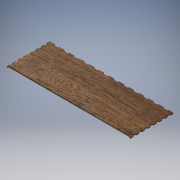
# Autodesk Inventor part: tavolaBase
Saved by Autodesk Inventor 2018.3 (Build 223284000, 284)
## iProperties
Created: 2019-03-04
Part Number: tavolaBase
Material: Generico
Document SubType Name: Modeling
Designer: AlfyPc
Density: 1 g/cm^3
Appearance: Frassino bianco - Giava
Author: AlfyPc
Autodesk Inventor part; units mm, degrees
(part 1 of 2)
ref_plane "YZ Plane" through (0, 0, 0) normal (1, 0, 0) x (0, 1, 0)
ref_plane "XZ Plane" through (0, 0, 0) normal (0, 1, 0) x (-1, 0, 0)
ref_plane "XY Plane" through (0, 0, 0) normal (0, 0, 1) x (1, 0, 0)
sketch "Schizzo1" plane through (0, 0, 0) normal (0, 0, 1) x (1, 0, 0)
  line L0 (233.5, -78.5) -> (-233.5, -78.5)
  line L1 (-233.5, -78.5) -> (-233.5, 78.5)
  line L2 (-233.5, 78.5) -> (233.5, 78.5)
  line L3 (233.5, 78.5) -> (233.5, -78.5)
  line L4 (233.5, -78.5) -> (-233.5, 78.5) construction
  line L5 (-233.5, -78.5) -> (233.5, 78.5) construction
  point P0 (0, 0)
  dimension "d0" = 467
  dimension "d1" = 157
  constraints: 12 end point, 2 midpoint, 2 parallel, 1 horizontal, 1 perpendicular
  measures "d0" distance of L0.start L0.end
  measures "d1" distance of L0.end L1.end
extrude "Estrusione1" add sketch "Schizzo1" against normal blind 4
sketch "Schizzo3" plane through (0, 0, 0) normal (0, 0, 1) x (1, 0, 0)
  line L0 (233.5, -78.5) -> (-233.5, -78.5) projected
  line L1 (233.5, 78.5) -> (233.5, -78.5) projected
  line L2 (-233.5, 78.5) -> (233.5, 78.5) projected
  line L3 (-233.5, -78.5) -> (-233.5, 78.5) projected
  line L4 (-237.5, -82.5) -> (237.5, -82.5) construction
  line L5 (237.5, -82.5) -> (237.5, 82.5) construction
  line L6 (237.5, 82.5) -> (-237.5, 82.5) construction
  line L7 (-237.5, 82.5) -> (-237.5, -82.5) construction
  line L8 (237.5, -82.5) -> (218.5, -82.5)
  line L9 (218.5, -82.5) -> (218.5, -78.5)
  line L10 (218.5, -78.5) -> (237.5, -78.5)
  line L11 (237.5, -78.5) -> (237.5, -82.5)
  line L12 (237.5, 82.5) -> (218.5, 82.5)
  line L13 (218.5, 82.5) -> (218.5, 78.5)
  line L14 (218.5, 78.5) -> (237.5, 78.5)
  line L15 (237.5, 78.5) -> (237.5, 82.5)
  line L16 (237.5, -82.5) -> (233.5, -82.5)
  line L17 (233.5, -82.5) -> (233.5, -71.5)
  line L18 (233.5, -71.5) -> (237.5, -71.5)
  line L19 (237.5, -71.5) -> (237.5, -82.5)
  line L20 (-237.5, -82.5) -> (-233.5, -82.5)
  line L21 (-233.5, -82.5) -> (-233.5, -71.5)
  line L22 (-233.5, -71.5) -> (-237.5, -71.5)
  line L23 (-237.5, -71.5) -> (-237.5, -82.5)
  line L24 (218.5, -78.5) -> (218.5, -82.5)
  line L25 (218.5, -82.5) -> (214.5, -82.5)
  line L26 (199.5, -82.5) -> (199.5, -78.5)
  line L27 (199.5, -78.5) -> (218.5, -78.5)
  line L28 (218.5, -82.5) -> (199.5, -82.5)
  line L29 (199.5, 82.5) -> (199.5, 78.5)
  line L30 (199.5, 78.5) -> (218.5, 78.5)
  line L31 (218.5, 78.5) -> (218.5, 82.5)
  line L32 (218.5, 82.5) -> (199.5, 82.5)
  line L33 (199.5, -78.5) -> (199.5, -82.5)
  line L34 (199.5, -82.5) -> (195.5, -82.5)
  line L35 (180.5, -82.5) -> (180.5, -78.5)
  line L36 (180.5, -78.5) -> (199.5, -78.5)
  line L37 (199.5, -82.5) -> (180.5, -82.5)
  line L38 (180.5, 82.5) -> (180.5, 78.5)
  line L39 (180.5, 78.5) -> (199.5, 78.5)
  line L40 (199.5, 78.5) -> (199.5, 82.5)
  line L41 (199.5, 82.5) -> (180.5, 82.5)
  line L42 (180.5, -78.5) -> (180.5, -82.5)
  line L43 (180.5, -82.5) -> (176.5, -82.5)
  line L44 (161.5, -82.5) -> (161.5, -78.5)
  line L45 (161.5, -78.5) -> (180.5, -78.5)
  line L46 (180.5, -82.5) -> (161.5, -82.5)
  line L47 (161.5, 82.5) -> (161.5, 78.5)
  line L48 (161.5, 78.5) -> (180.5, 78.5)
  line L49 (180.5, 78.5) -> (180.5, 82.5)
  line L50 (180.5, 82.5) -> (161.5, 82.5)
  line L51 (161.5, -78.5) -> (161.5, -82.5)
  line L52 (161.5, -82.5) -> (157.5, -82.5)
  line L53 (142.5, -82.5) -> (142.5, -78.5)
  line L54 (142.5, -78.5) -> (161.5, -78.5)
  line L55 (161.5, -82.5) -> (142.5, -82.5)
  line L56 (142.5, 82.5) -> (142.5, 78.5)
  line L57 (142.5, 78.5) -> (161.5, 78.5)
  line L58 (161.5, 78.5) -> (161.5, 82.5)
  line L59 (161.5, 82.5) -> (142.5, 82.5)
  line L60 (142.5, -78.5) -> (142.5, -82.5)
  line L61 (142.5, -82.5) -> (138.5, -82.5)
  line L62 (123.5, -82.5) -> (123.5, -78.5)
  line L63 (123.5, -78.5) -> (142.5, -78.5)
  line L64 (142.5, -82.5) -> (123.5, -82.5)
  line L65 (123.5, 82.5) -> (123.5, 78.5)
  line L66 (123.5, 78.5) -> (142.5, 78.5)
  line L67 (142.5, 78.5) -> (142.5, 82.5)
  line L68 (142.5, 82.5) -> (123.5, 82.5)
  line L69 (123.5, -78.5) -> (123.5, -82.5)
  line L70 (123.5, -82.5) -> (119.5, -82.5)
  line L71 (104.5, -82.5) -> (104.5, -78.5)
  line L72 (104.5, -78.5) -> (123.5, -78.5)
  line L73 (123.5, -82.5) -> (104.5, -82.5)
  line L74 (104.5, 82.5) -> (104.5, 78.5)
  line L75 (104.5, 78.5) -> (123.5, 78.5)
  line L76 (123.5, 78.5) -> (123.5, 82.5)
  line L77 (123.5, 82.5) -> (104.5, 82.5)
  line L78 (104.5, -78.5) -> (104.5, -82.5)
  line L79 (104.5, -82.5) -> (100.5, -82.5)
  line L80 (85.5, -82.5) -> (85.5, -78.5)
  line L81 (85.5, -78.5) -> (104.5, -78.5)
  line L82 (104.5, -82.5) -> (85.5, -82.5)
  line L83 (85.5, 82.5) -> (85.5, 78.5)
  line L84 (85.5, 78.5) -> (104.5, 78.5)
  line L85 (104.5, 78.5) -> (104.5, 82.5)
  line L86 (104.5, 82.5) -> (85.5, 82.5)
  line L87 (85.5, -78.5) -> (85.5, -82.5)
  line L88 (85.5, -82.5) -> (81.5, -82.5)
  line L89 (66.5, -82.5) -> (66.5, -78.5)
  line L90 (66.5, -78.5) -> (85.5, -78.5)
  line L91 (85.5, -82.5) -> (66.5, -82.5)
  line L92 (66.5, 82.5) -> (66.5, 78.5)
  line L93 (66.5, 78.5) -> (85.5, 78.5)
  line L94 (85.5, 78.5) -> (85.5, 82.5)
  line L95 (85.5, 82.5) -> (66.5, 82.5)
  line L96 (66.5, -78.5) -> (66.5, -82.5)
  line L97 (66.5, -82.5) -> (62.5, -82.5)
  line L98 (47.5, -82.5) -> (47.5, -78.5)
  line L99 (47.5, -78.5) -> (66.5, -78.5)
  line L100 (66.5, -82.5) -> (47.5, -82.5)
  line L101 (47.5, 82.5) -> (47.5, 78.5)
  line L102 (47.5, 78.5) -> (66.5, 78.5)
  line L103 (66.5, 78.5) -> (66.5, 82.5)
  line L104 (66.5, 82.5) -> (47.5, 82.5)
  line L105 (47.5, -78.5) -> (47.5, -82.5)
  line L106 (47.5, -82.5) -> (43.5, -82.5)
  line L107 (28.5, -82.5) -> (28.5, -78.5)
  line L108 (28.5, -78.5) -> (47.5, -78.5)
  line L109 (47.5, -82.5) -> (28.5, -82.5)
  line L110 (28.5, 82.5) -> (28.5, 78.5)
  line L111 (28.5, 78.5) -> (47.5, 78.5)
  line L112 (47.5, 78.5) -> (47.5, 82.5)
  line L113 (47.5, 82.5) -> (28.5, 82.5)
  line L114 (28.5, -78.5) -> (28.5, -82.5)
  line L115 (28.5, -82.5) -> (24.5, -82.5)
  line L116 (9.5, -82.5) -> (9.5, -78.5)
  line L117 (9.5, -78.5) -> (28.5, -78.5)
  line L118 (28.5, -82.5) -> (9.5, -82.5)
  line L119 (9.5, 82.5) -> (9.5, 78.5)
  line L120 (9.5, 78.5) -> (28.5, 78.5)
  line L121 (28.5, 78.5) -> (28.5, 82.5)
  line L122 (28.5, 82.5) -> (9.5, 82.5)
  line L123 (9.5, -78.5) -> (9.5, -82.5)
  line L124 (9.5, -82.5) -> (5.5, -82.5)
  line L125 (-9.5, -82.5) -> (-9.5, -78.5)
  line L126 (-9.5, -78.5) -> (9.5, -78.5)
  line L127 (9.5, -82.5) -> (-9.5, -82.5)
  line L128 (-9.5, 82.5) -> (-9.5, 78.5)
  line L129 (-9.5, 78.5) -> (9.5, 78.5)
  line L130 (9.5, 78.5) -> (9.5, 82.5)
  line L131 (9.5, 82.5) -> (-9.5, 82.5)
  line L132 (-9.5, -78.5) -> (-9.5, -82.5)
  line L133 (-9.5, -82.5) -> (-13.5, -82.5)
  line L134 (-28.5, -82.5) -> (-28.5, -78.5)
  line L135 (-28.5, -78.5) -> (-9.5, -78.5)
  line L136 (-9.5, -82.5) -> (-28.5, -82.5)
  line L137 (-28.5, 82.5) -> (-28.5, 78.5)
  line L138 (-28.5, 78.5) -> (-9.5, 78.5)
  line L139 (-9.5, 78.5) -> (-9.5, 82.5)
  line L140 (-9.5, 82.5) -> (-28.5, 82.5)
  line L141 (-28.5, -78.5) -> (-28.5, -82.5)
  line L142 (-28.5, -82.5) -> (-32.5, -82.5)
  line L143 (-47.5, -82.5) -> (-47.5, -78.5)
  line L144 (-47.5, -78.5) -> (-28.5, -78.5)
  line L145 (-28.5, -82.5) -> (-47.5, -82.5)
  line L146 (-47.5, 82.5) -> (-47.5, 78.5)
  line L147 (-47.5, 78.5) -> (-28.5, 78.5)
  line L148 (-28.5, 78.5) -> (-28.5, 82.5)
  line L149 (-28.5, 82.5) -> (-47.5, 82.5)
  line L150 (-47.5, -78.5) -> (-47.5, -82.5)
  line L151 (-47.5, -82.5) -> (-51.5, -82.5)
  line L152 (-66.5, -82.5) -> (-66.5, -78.5)
  line L153 (-66.5, -78.5) -> (-47.5, -78.5)
  line L154 (-47.5, -82.5) -> (-66.5, -82.5)
  line L155 (-66.5, 82.5) -> (-66.5, 78.5)
  line L156 (-66.5, 78.5) -> (-47.5, 78.5)
  line L157 (-47.5, 78.5) -> (-47.5, 82.5)
  line L158 (-47.5, 82.5) -> (-66.5, 82.5)
  line L159 (-66.5, -78.5) -> (-66.5, -82.5)
  line L160 (-66.5, -82.5) -> (-70.5, -82.5)
  line L161 (-85.5, -82.5) -> (-85.5, -78.5)
  line L162 (-85.5, -78.5) -> (-66.5, -78.5)
  line L163 (-66.5, -82.5) -> (-85.5, -82.5)
  line L164 (-85.5, 82.5) -> (-85.5, 78.5)
  line L165 (-85.5, 78.5) -> (-66.5, 78.5)
  line L166 (-66.5, 78.5) -> (-66.5, 82.5)
  line L167 (-66.5, 82.5) -> (-85.5, 82.5)
  line L168 (-85.5, -78.5) -> (-85.5, -82.5)
  line L169 (-85.5, -82.5) -> (-89.5, -82.5)
  line L170 (-104.5, -82.5) -> (-104.5, -78.5)
  line L171 (-104.5, -78.5) -> (-85.5, -78.5)
  line L172 (-85.5, -82.5) -> (-104.5, -82.5)
  line L173 (-104.5, 82.5) -> (-104.5, 78.5)
  line L174 (-104.5, 78.5) -> (-85.5, 78.5)
  line L175 (-85.5, 78.5) -> (-85.5, 82.5)
  line L176 (-85.5, 82.5) -> (-104.5, 82.5)
  line L177 (-104.5, -78.5) -> (-104.5, -82.5)
  line L178 (-104.5, -82.5) -> (-108.5, -82.5)
  line L179 (-123.5, -82.5) -> (-123.5, -78.5)
  line L180 (-123.5, -78.5) -> (-104.5, -78.5)
  line L181 (-104.5, -82.5) -> (-123.5, -82.5)
  line L182 (-123.5, 82.5) -> (-123.5, 78.5)
  line L183 (-123.5, 78.5) -> (-104.5, 78.5)
  line L184 (-104.5, 78.5) -> (-104.5, 82.5)
  line L185 (-104.5, 82.5) -> (-123.5, 82.5)
  line L186 (-123.5, -78.5) -> (-123.5, -82.5)
  line L187 (-123.5, -82.5) -> (-127.5, -82.5)
  line L188 (-142.5, -82.5) -> (-142.5, -78.5)
  line L189 (-142.5, -78.5) -> (-123.5, -78.5)
  line L190 (-123.5, -82.5) -> (-142.5, -82.5)
  line L191 (-142.5, 82.5) -> (-142.5, 78.5)
  line L192 (-142.5, 78.5) -> (-123.5, 78.5)
  line L193 (-123.5, 78.5) -> (-123.5, 82.5)
  line L194 (-123.5, 82.5) -> (-142.5, 82.5)
  line L195 (-142.5, -78.5) -> (-142.5, -82.5)
  line L196 (-142.5, -82.5) -> (-146.5, -82.5)
  line L197 (-161.5, -82.5) -> (-161.5, -78.5)
  line L198 (-161.5, -78.5) -> (-142.5, -78.5)
  line L199 (-142.5, -82.5) -> (-161.5, -82.5)
  line L200 (-161.5, 82.5) -> (-161.5, 78.5)
  line L201 (-161.5, 78.5) -> (-142.5, 78.5)
  line L202 (-142.5, 78.5) -> (-142.5, 82.5)
  line L203 (-142.5, 82.5) -> (-161.5, 82.5)
  line L204 (-161.5, -78.5) -> (-161.5, -82.5)
  line L205 (-161.5, -82.5) -> (-165.5, -82.5)
  line L206 (-180.5, -82.5) -> (-180.5, -78.5)
  line L207 (-180.5, -78.5) -> (-161.5, -78.5)
  line L208 (-161.5, -82.5) -> (-180.5, -82.5)
  line L209 (-180.5, 82.5) -> (-180.5, 78.5)
  line L210 (-180.5, 78.5) -> (-161.5, 78.5)
  line L211 (-161.5, 78.5) -> (-161.5, 82.5)
  line L212 (-161.5, 82.5) -> (-180.5, 82.5)
  line L213 (-180.5, -78.5) -> (-180.5, -82.5)
  line L214 (-180.5, -82.5) -> (-184.5, -82.5)
  line L215 (-199.5, -82.5) -> (-199.5, -78.5)
  line L216 (-199.5, -78.5) -> (-180.5, -78.5)
  line L217 (-180.5, -82.5) -> (-199.5, -82.5)
  line L218 (-199.5, 82.5) -> (-199.5, 78.5)
  line L219 (-199.5, 78.5) -> (-180.5, 78.5)
  line L220 (-180.5, 78.5) -> (-180.5, 82.5)
  line L221 (-180.5, 82.5) -> (-199.5, 82.5)
  line L222 (-199.5, -78.5) -> (-199.5, -82.5)
  line L223 (-199.5, -82.5) -> (-203.5, -82.5)
  line L224 (-218.5, -82.5) -> (-218.5, -78.5)
  line L225 (-218.5, -78.5) -> (-199.5, -78.5)
  line L226 (-199.5, -82.5) -> (-218.5, -82.5)
  line L227 (-218.5, 82.5) -> (-218.5, 78.5)
  line L228 (-218.5, 78.5) -> (-199.5, 78.5)
  line L229 (-199.5, 78.5) -> (-199.5, 82.5)
  line L230 (-199.5, 82.5) -> (-218.5, 82.5)
  line L231 (-218.5, -78.5) -> (-218.5, -82.5)
  line L232 (-218.5, -82.5) -> (-222.5, -82.5)
  line L233 (-237.5, -82.5) -> (-237.5, -78.5)
  line L234 (-237.5, -78.5) -> (-218.5, -78.5)
  line L235 (-218.5, -82.5) -> (-237.5, -82.5)
  line L236 (-237.5, 82.5) -> (-237.5, 78.5)
  line L237 (-237.5, 78.5) -> (-218.5, 78.5)
  line L238 (-218.5, 78.5) -> (-218.5, 82.5)
  line L239 (-218.5, 82.5) -> (-237.5, 82.5)
  line L240 (237.5, -67.5) -> (237.5, -71.5)
  line L241 (237.5, -71.5) -> (233.5, -71.5)
  line L242 (233.5, -60.5) -> (237.5, -60.5)
  line L243 (237.5, -60.5) -> (237.5, -71.5)
  line L244 (233.5, -71.5) -> (233.5, -60.5)
  line L245 (-237.5, -71.5) -> (-233.5, -71.5)
  line L246 (-233.5, -71.5) -> (-233.5, -60.5)
  line L247 (-233.5, -60.5) -> (-237.5, -60.5)
  line L248 (-237.5, -60.5) -> (-237.5, -71.5)
  line L249 (-237.5, -71.5) -> (-237.5, -67.5)
  line L250 (237.5, -56.5) -> (237.5, -60.5)
  line L251 (237.5, -60.5) -> (233.5, -60.5)
  line L252 (233.5, -49.5) -> (237.5, -49.5)
  line L253 (237.5, -49.5) -> (237.5, -60.5)
  line L254 (233.5, -60.5) -> (233.5, -49.5)
  line L255 (-237.5, -60.5) -> (-233.5, -60.5)
  line L256 (-233.5, -60.5) -> (-233.5, -49.5)
  line L257 (-233.5, -49.5) -> (-237.5, -49.5)
  line L258 (-237.5, -49.5) -> (-237.5, -60.5)
  line L259 (-237.5, -60.5) -> (-237.5, -56.5)
  line L260 (237.5, -45.5) -> (237.5, -49.5)
  line L261 (237.5, -49.5) -> (233.5, -49.5)
  line L262 (233.5, -38.5) -> (237.5, -38.5)
  line L263 (237.5, -38.5) -> (237.5, -49.5)
  line L264 (233.5, -49.5) -> (233.5, -38.5)
  line L265 (-237.5, -49.5) -> (-233.5, -49.5)
  line L266 (-233.5, -49.5) -> (-233.5, -38.5)
  line L267 (-233.5, -38.5) -> (-237.5, -38.5)
  line L268 (-237.5, -38.5) -> (-237.5, -49.5)
  line L269 (-237.5, -49.5) -> (-237.5, -45.5)
  line L270 (237.5, -34.5) -> (237.5, -38.5)
  line L271 (237.5, -38.5) -> (233.5, -38.5)
  line L272 (233.5, -27.5) -> (237.5, -27.5)
  line L273 (237.5, -27.5) -> (237.5, -38.5)
  line L274 (233.5, -38.5) -> (233.5, -27.5)
  line L275 (-237.5, -38.5) -> (-233.5, -38.5)
  line L276 (-233.5, -38.5) -> (-233.5, -27.5)
  line L277 (-233.5, -27.5) -> (-237.5, -27.5)
  line L278 (-237.5, -27.5) -> (-237.5, -38.5)
  line L279 (-237.5, -38.5) -> (-237.5, -34.5)
  line L280 (237.5, -23.5) -> (237.5, -27.5)
  line L281 (237.5, -27.5) -> (233.5, -27.5)
  line L282 (233.5, -16.5) -> (237.5, -16.5)
  line L283 (237.5, -16.5) -> (237.5, -27.5)
  line L284 (233.5, -27.5) -> (233.5, -16.5)
  line L285 (-237.5, -27.5) -> (-233.5, -27.5)
  line L286 (-233.5, -27.5) -> (-233.5, -16.5)
  line L287 (-233.5, -16.5) -> (-237.5, -16.5)
  line L288 (-237.5, -16.5) -> (-237.5, -27.5)
  line L289 (-237.5, -27.5) -> (-237.5, -23.5)
  line L290 (237.5, -12.5) -> (237.5, -16.5)
  line L291 (237.5, -16.5) -> (233.5, -16.5)
  line L292 (233.5, -5.5) -> (237.5, -5.5)
  line L293 (237.5, -5.5) -> (237.5, -16.5)
  line L294 (233.5, -16.5) -> (233.5, -5.5)
  line L295 (-237.5, -16.5) -> (-233.5, -16.5)
  line L296 (-233.5, -16.5) -> (-233.5, -5.5)
  line L297 (-233.5, -5.5) -> (-237.5, -5.5)
  line L298 (-237.5, -5.5) -> (-237.5, -16.5)
  line L299 (-237.5, -16.5) -> (-237.5, -12.5)
  line L300 (237.5, -1.5) -> (237.5, -5.5)
  line L301 (237.5, -5.5) -> (233.5, -5.5)
  line L302 (233.5, 5.5) -> (237.5, 5.5)
  line L303 (237.5, 5.5) -> (237.5, -5.5)
  line L304 (233.5, -5.5) -> (233.5, 5.5)
  line L305 (-237.5, -5.5) -> (-233.5, -5.5)
  line L306 (-233.5, -5.5) -> (-233.5, 5.5)
  line L307 (-233.5, 5.5) -> (-237.5, 5.5)
  line L308 (-237.5, 5.5) -> (-237.5, -5.5)
  line L309 (-237.5, -5.5) -> (-237.5, -1.5)
  line L310 (237.5, 9.5) -> (237.5, 5.5)
  line L311 (237.5, 5.5) -> (233.5, 5.5)
  line L312 (233.5, 16.5) -> (237.5, 16.5)
  line L313 (237.5, 16.5) -> (237.5, 5.5)
  line L314 (233.5, 5.5) -> (233.5, 16.5)
  line L315 (-237.5, 5.5) -> (-233.5, 5.5)
  line L316 (-233.5, 5.5) -> (-233.5, 16.5)
  line L317 (-233.5, 16.5) -> (-237.5, 16.5)
  line L318 (-237.5, 16.5) -> (-237.5, 5.5)
  line L319 (-237.5, 5.5) -> (-237.5, 9.5)
  line L320 (237.5, 20.5) -> (237.5, 16.5)
  line L321 (237.5, 16.5) -> (233.5, 16.5)
  line L322 (233.5, 27.5) -> (237.5, 27.5)
  line L323 (237.5, 27.5) -> (237.5, 16.5)
  line L324 (233.5, 16.5) -> (233.5, 27.5)
  line L325 (-237.5, 16.5) -> (-233.5, 16.5)
  line L326 (-233.5, 16.5) -> (-233.5, 27.5)
  line L327 (-233.5, 27.5) -> (-237.5, 27.5)
  line L328 (-237.5, 27.5) -> (-237.5, 16.5)
  line L329 (-237.5, 16.5) -> (-237.5, 20.5)
  line L330 (237.5, 31.5) -> (237.5, 27.5)
  line L331 (237.5, 27.5) -> (233.5, 27.5)
  line L332 (233.5, 38.5) -> (237.5, 38.5)
  line L333 (237.5, 38.5) -> (237.5, 27.5)
  line L334 (233.5, 27.5) -> (233.5, 38.5)
  line L335 (-237.5, 27.5) -> (-233.5, 27.5)
  line L336 (-233.5, 27.5) -> (-233.5, 38.5)
  line L337 (-233.5, 38.5) -> (-237.5, 38.5)
  line L338 (-237.5, 38.5) -> (-237.5, 27.5)
  line L339 (-237.5, 27.5) -> (-237.5, 31.5)
  line L340 (237.5, 42.5) -> (237.5, 38.5)
  line L341 (237.5, 38.5) -> (233.5, 38.5)
  line L342 (233.5, 49.5) -> (237.5, 49.5)
  line L343 (237.5, 49.5) -> (237.5, 38.5)
  line L344 (233.5, 38.5) -> (233.5, 49.5)
  line L345 (-237.5, 38.5) -> (-233.5, 38.5)
  line L346 (-233.5, 38.5) -> (-233.5, 49.5)
  line L347 (-233.5, 49.5) -> (-237.5, 49.5)
  line L348 (-237.5, 49.5) -> (-237.5, 38.5)
  line L349 (-237.5, 38.5) -> (-237.5, 42.5)
  line L350 (237.5, 53.5) -> (237.5, 49.5)
  line L351 (237.5, 49.5) -> (233.5, 49.5)
  line L352 (233.5, 60.5) -> (237.5, 60.5)
  line L353 (237.5, 60.5) -> (237.5, 49.5)
  line L354 (233.5, 49.5) -> (233.5, 60.5)
  line L355 (-237.5, 49.5) -> (-233.5, 49.5)
  line L356 (-233.5, 49.5) -> (-233.5, 60.5)
  line L357 (-233.5, 60.5) -> (-237.5, 60.5)
  line L358 (-237.5, 60.5) -> (-237.5, 49.5)
  line L359 (-237.5, 49.5) -> (-237.5, 53.5)
  line L360 (237.5, 64.5) -> (237.5, 60.5)
  line L361 (237.5, 60.5) -> (233.5, 60.5)
  line L362 (233.5, 71.5) -> (237.5, 71.5)
  line L363 (237.5, 71.5) -> (237.5, 60.5)
  line L364 (233.5, 60.5) -> (233.5, 71.5)
  line L365 (-237.5, 60.5) -> (-233.5, 60.5)
  line L366 (-233.5, 60.5) -> (-233.5, 71.5)
  line L367 (-233.5, 71.5) -> (-237.5, 71.5)
  line L368 (-237.5, 71.5) -> (-237.5, 60.5)
  line L369 (-237.5, 60.5) -> (-237.5, 64.5)
  line L370 (237.5, 75.5) -> (237.5, 71.5)
  line L371 (237.5, 71.5) -> (233.5, 71.5)
  line L372 (233.5, 82.5) -> (237.5, 82.5)
  line L373 (237.5, 82.5) -> (237.5, 71.5)
  line L374 (233.5, 71.5) -> (233.5, 82.5)
  line L375 (-237.5, 71.5) -> (-233.5, 71.5)
  line L376 (-233.5, 71.5) -> (-233.5, 82.5)
  line L377 (-233.5, 82.5) -> (-237.5, 82.5)
  line L378 (-237.5, 82.5) -> (-237.5, 71.5)
  line L379 (-237.5, 71.5) -> (-237.5, 75.5)
  point P0 (0, 0)
  point P1 (214.5, -78.5)
  point P2 (214.5, 78.5)
  point P3 (195.5, -78.5)
  point P4 (195.5, 78.5)
  point P5 (176.5, -78.5)
  point P6 (176.5, 78.5)
  point P7 (157.5, -78.5)
  point P8 (157.5, 78.5)
  point P9 (138.5, -78.5)
  point P10 (138.5, 78.5)
  point P11 (119.5, -78.5)
  point P12 (119.5, 78.5)
  point P13 (100.5, -78.5)
  point P14 (100.5, 78.5)
  point P15 (81.5, -78.5)
  point P16 (81.5, 78.5)
  point P17 (62.5, -78.5)
  point P18 (62.5, 78.5)
  point P19 (43.5, -78.5)
  point P20 (43.5, 78.5)
  point P21 (24.5, -78.5)
  point P22 (24.5, 78.5)
  point P23 (5.5, -78.5)
  point P24 (5.5, 78.5)
  point P25 (-13.5, -78.5)
  point P26 (-13.5, 78.5)
  point P27 (-32.5, -78.5)
  point P28 (-32.5, 78.5)
  point P29 (-51.5, -78.5)
  point P30 (-51.5, 78.5)
  point P31 (-70.5, -78.5)
  point P32 (-70.5, 78.5)
  point P33 (-89.5, -78.5)
  point P34 (-89.5, 78.5)
  point P35 (-108.5, -78.5)
  point P36 (-108.5, 78.5)
  point P37 (-127.5, -78.5)
  point P38 (-127.5, 78.5)
  point P39 (-146.5, -78.5)
  point P40 (-146.5, 78.5)
  point P41 (-165.5, -78.5)
  point P42 (-165.5, 78.5)
  point P43 (-184.5, -78.5)
  point P44 (-184.5, 78.5)
  point P45 (-203.5, -78.5)
  point P46 (-203.5, 78.5)
  point P47 (-222.5, -78.5)
  point P48 (-222.5, 78.5)
  point P49 (233.5, -67.5)
  point P50 (-233.5, -67.5)
  point P51 (233.5, -56.5)
  point P52 (-233.5, -56.5)
  point P53 (233.5, -45.5)
  point P54 (-233.5, -45.5)
  point P55 (233.5, -34.5)
  point P56 (-233.5, -34.5)
  point P57 (233.5, -23.5)
  point P58 (-233.5, -23.5)
  point P59 (233.5, -12.5)
  point P60 (-233.5, -12.5)
  point P61 (233.5, -1.5)
  point P62 (-233.5, -1.5)
  point P63 (233.5, 9.5)
  point P64 (-233.5, 9.5)
  point P65 (233.5, 20.5)
  point P66 (-233.5, 20.5)
  point P67 (233.5, 31.5)
  point P68 (-233.5, 31.5)
  point P69 (233.5, 42.5)
  point P70 (-233.5, 42.5)
  point P71 (233.5, 53.5)
  point P72 (-233.5, 53.5)
  point P73 (233.5, 64.5)
  point P74 (-233.5, 64.5)
  point P75 (233.5, 75.5)
  point P76 (-233.5, 75.5)
  dimension "d28" = 4
  dimension "d29" = 475
  dimension "d30" = 165
  dimension "d31" = 19
  dimension "d32" = 4
  dimension "d33" = 19
  dimension "d34" = 4
  dimension "d35" = 4
  dimension "d36" = 11
  dimension "d37" = 4
  dimension "d38" = 11
  dimension "d41" = 19
  dimension "d48" = 11
  constraints: 752 end point, 8 parallel, 5 horizontal, 4 perpendicular, 1 vertical, 805 other
  measures "d28" distance between parallel lines of L0 L4
  measures "d29" distance of L4.start L4.end
  measures "d30" distance of L4.end L5.end
  measures "d31" distance of L9.end L10.end
  measures "d32" distance of L8.end L9.end
  measures "d33" distance of L14.end L13.end
  measures "d34" distance of L13.end L12.end
  measures "d35" distance of L17.end L18.end
  measures "d36" distance of L16.end L17.end
  measures "d37" distance of L22.end L21.end
  measures "d38" distance of L21.end L20.end
  measures "d41" distance of L10.end L24.start
  measures "d48" distance of L0.start point (233.5, -67.5)
extrude "Estrusione2" add sketch "Schizzo3" against normal up to surface (4 mm away) contours L1 L18 L19 L10 | L10 L11 L8 L17 | L1 L252 L253 L250 L242 | L1 L272 L273 L270 L262 | L1 L292 L293 L290 L282 | L1 L312 L313 L310 L302 | L1 L332 L333 L330 L322 | L1 L352 L353 L350 L342 | L1 L14 L373 L370 L362 | L374 L12 L15 L14 | L2 L13 L12 L374 | L2 L38 L41 L29 | L2 L56 L59 L47 | L2 L74 L77 L65 | L2 L92 L95 L83 | L234 L23 L22 L3 | L21 L20 L23 L234 | L2 L110 L113 L101 | L247 L258 L257 L3 | L2 L128 L131 L119 | L267 L278 L277 L3 | L2 L146 L149 L137 | L287 L298 L297 L3 | L2 L164 L167 L155 | L307 L318 L317 L3 | L2 L182 L185 L173 | L327 L338 L337 L3 | L2 L200 L203 L191 | L347 L358 L357 L3 | L2 L218 L221 L209 | L367 L378 L237 L3 | L2 L376 L239 L227 | L237 L236 L239 L376
sketch "Schizzo4" plane through (0, 0, 0) normal (0, 0, 1) x (1, 0, 0)
  circle A0 centre (29.075, -39.395) radius 1.5
  circle A1 centre (29.075, 41.885) radius 1.5
  circle A2 centre (-135.39, -38.76) radius 1.5
  circle A3 centre (-173.97, 42.5) radius 1.375
  circle A4 centre (-222.97, 42.5) radius 1.375
  circle A5 centre (-173.97, -15.5) radius 1.375
  circle A6 centre (-222.97, -15.5) radius 1.375
  point P0 (0, 0)
extrude "Estrusione3" cut sketch "Schizzo4" against normal blind 10
sketch "Schizzo5" plane through (0, 0, 0) normal (0, 0, 1) x (1, 0, 0)
  line L0 (-55.35, 78.5) -> (-58.65, 78.5) projected
  line L1 (-233.5, -64.35) -> (-233.5, -67.65) projected
  line L2 (-233.5, -71.5) -> (-233.5, -60.5) construction
  line L3 (-233.5, -66) -> (-220.5, -66) construction
  circle A0 centre (-220.5, -66) radius 1.65
  line L4 (-66.5, 78.5) -> (-47.5, 78.5) construction
  line L5 (-57, 78.5) -> (-57, 65.5) construction
  circle A1 centre (-57, 65.5) radius 1.65
  line L6 (233.5, -67.65) -> (233.5, -64.35) projected
  line L7 (233.5, -60.5) -> (233.5, -71.5) projected
  line L8 (233.5, -66) -> (220.5, -66) construction
  circle A2 centre (220.5, -66) radius 1.65
  dimension "d75" = 13
  dimension "d76" = 3.3
  dimension "d77" = 13
  dimension "d78" = 3.3
  dimension "d79" = 13
  dimension "d80" = 3.3
  constraints: 6 end point, 3 centre point, 3 coincident, 3 midpoint, 1 horizontal, 1 perpendicular, 1 vertical
  measures "d75" distance of L3.start L3.end
  measures "d76" diameter of A0
  measures "d77" distance of L5.start L5.end
  measures "d78" diameter of A1
  measures "d79" distance of L8.start L8.end
  measures "d80" diameter of A2
extrude "Estrusione4" cut sketch "Schizzo5" against normal blind 10
sketch "Schizzo6" plane through (0, 0, 0) normal (0, 0, 1) x (1, 0, 0)
  line L0 (-139.4893, -62.5844) -> (-76.5866, -62.5844) construction
  line L1 (-76.5866, -62.5844) -> (-76.5866, -76.1722) construction
  line L2 (-76.5866, -76.1722) -> (-139.4893, -76.1722) construction
  line L3 (-139.4893, -76.1722) -> (-139.4893, -62.5844) construction
  line L4 (-164.8687, -21.1575) -> (-142, -21.1575)
  line L5 (-142, -21.1575) -> (-142, -69)
  line L6 (-142, -69) -> (-164.8687, -69)
  line L7 (-164.8687, -69) -> (-164.8687, -21.1575)
  spline S0 degree 2 poles (-136.5836, -64.8733) (-136.5836, -65.3231) (-137.2145, -65.8098) (-137.7974, -65.8098) knots 0 0 0 1 2 2 2
  line L8 (-137.7974, -65.8098) -> (-139.1894, -65.8098)
  line L9 (-139.1894, -65.8098) -> (-139.1894, -62.7598)
  line L10 (-139.1894, -62.7598) -> (-137.8936, -62.7598)
  spline S1 degree 2 poles (-137.8936, -62.7598) (-136.6798, -62.7598) (-136.6798, -63.4982) knots 0 0 0 1 1 1
  spline S2 degree 2 poles (-136.6798, -63.4982) (-136.6798, -63.6567) (-136.8326, -63.9226) (-137.1466, -64.1235) (-137.3334, -64.1603) knots 0 0 0 1 2 3 3 3
  line L11 (-137.3334, -64.1603) -> (-137.3334, -64.1688)
  spline S3 degree 2 poles (-137.3334, -64.1688) (-137.1155, -64.1942) (-136.7703, -64.4008) (-136.5836, -64.7092) (-136.5836, -64.8733) knots 0 0 0 1 2 3 3 3
  spline S4 degree 2 poles (-137.5597, -64.8705) (-137.5597, -64.7375) (-137.7521, -64.5677) (-137.9077, -64.5677) knots 0 0 0 1 2 2 2
  line L12 (-137.9077, -64.5677) -> (-138.2699, -64.5677)
  line L13 (-138.2699, -64.5677) -> (-138.2699, -65.1902)
  line L14 (-138.2699, -65.1902) -> (-137.9643, -65.1902)
  spline S5 degree 2 poles (-137.9643, -65.1902) (-137.7776, -65.1902) (-137.5597, -65.0176) (-137.5597, -64.8705) knots 0 0 0 1 2 2 2
  spline S6 degree 2 poles (-137.6559, -63.6567) (-137.6559, -63.3737) (-138.1001, -63.3737) knots 0 0 0 1 1 1
  line L15 (-138.1001, -63.3737) -> (-138.2699, -63.3737)
  line L16 (-138.2699, -63.3737) -> (-138.2699, -63.9509)
  line L17 (-138.2699, -63.9509) -> (-138.0039, -63.9509)
  spline S7 degree 2 poles (-138.0039, -63.9509) (-137.8511, -63.9509) (-137.6559, -63.7868) (-137.6559, -63.6567) knots 0 0 0 1 2 2 2
  spline S8 degree 2 poles (-133.8392, -64.6809) (-133.8392, -65.2326) (-134.5041, -65.8635) (-135.101, -65.8635) knots 0 0 0 1 2 2 2
  spline S9 degree 2 poles (-135.101, -65.8635) (-135.6952, -65.8635) (-136.3573, -65.2496) (-136.3573, -64.7064) knots 0 0 0 1 2 2 2
  spline S10 degree 2 poles (-136.3573, -64.7064) (-136.3573, -64.3612) (-136.046, -63.8491) (-135.4717, -63.5775) (-135.0982, -63.5775) knots 0 0 0 1 2 3 3 3
  spline S11 degree 2 poles (-135.0982, -63.5775) (-134.7106, -63.5775) (-134.1419, -63.8632) (-133.8392, -64.3697) (-133.8392, -64.6809) knots 0 0 0 1 2 3 3 3
  spline S12 degree 2 poles (-134.7587, -64.6865) (-134.7587, -64.2423) (-135.0982, -64.2423) knots 0 0 0 1 1 1
  spline S13 degree 2 poles (-135.0982, -64.2423) (-135.4377, -64.2423) (-135.4377, -64.7064) knots 0 0 0 1 1 1
  spline S14 degree 2 poles (-135.4377, -64.7064) (-135.4377, -65.1987) (-135.0926, -65.1987) knots 0 0 0 1 1 1
  spline S15 degree 2 poles (-135.0926, -65.1987) (-134.7587, -65.1987) (-134.7587, -64.6865) knots 0 0 0 1 1 1
  line L18 (-132.2915, -65.8098) -> (-132.2915, -65.4788)
  line L19 (-132.2915, -65.4788) -> (-132.3, -65.4788)
  spline S16 degree 2 poles (-132.3, -65.4788) (-132.5179, -65.8635) (-132.9649, -65.8635) knots 0 0 0 1 1 1
  spline S17 degree 2 poles (-132.9649, -65.8635) (-133.2733, -65.8635) (-133.6213, -65.4986) (-133.6213, -65.1902) knots 0 0 0 1 2 2 2
  spline S18 degree 2 poles (-133.6213, -65.1902) (-133.6213, -64.5479) (-132.8319, -64.4461) knots 0 0 0 1 1 1
  line L20 (-132.8319, -64.4461) -> (-132.2915, -64.3753)
  spline S19 degree 2 poles (-132.2915, -64.3753) (-132.2915, -64.2678) (-132.4839, -64.132) (-132.6452, -64.132) knots 0 0 0 1 2 2 2
  spline S20 degree 2 poles (-132.6452, -64.132) (-133.0102, -64.132) (-133.4176, -64.3414) knots 0 0 0 1 1 1
  line L21 (-133.4176, -64.3414) -> (-133.4176, -63.7529)
  spline S21 degree 2 poles (-133.4176, -63.7529) (-133.2422, -63.6765) (-132.7074, -63.5775) (-132.5179, -63.5775) knots 0 0 0 1 2 2 2
  spline S22 degree 2 poles (-132.5179, -63.5775) (-131.9633, -63.5775) (-131.4625, -64.0528) (-131.4625, -64.6073) knots 0 0 0 1 2 2 2
  line L22 (-131.4625, -64.6073) -> (-131.4625, -65.8098)
  line L23 (-131.4625, -65.8098) -> (-132.2915, -65.8098)
  spline S23 degree 2 poles (-132.8291, -65.0685) (-132.8291, -65.1562) (-132.7159, -65.2722) (-132.6112, -65.2722) knots 0 0 0 1 2 2 2
  spline S24 degree 2 poles (-132.6112, -65.2722) (-132.4698, -65.2722) (-132.2915, -65.06) (-132.2915, -64.8931) knots 0 0 0 1 2 2 2
  line L24 (-132.2915, -64.8931) -> (-132.2915, -64.811)
  line L25 (-132.2915, -64.811) -> (-132.5999, -64.8535)
  spline S25 degree 2 poles (-132.5999, -64.8535) (-132.8291, -64.8931) (-132.8291, -65.0685) knots 0 0 0 1 1 1
  spline S26 degree 2 poles (-129.417, -64.4064) (-129.4679, -64.3838) (-129.6433, -64.347) (-129.6999, -64.347) knots 0 0 0 1 2 2 2
  spline S27 degree 2 poles (-129.6999, -64.347) (-130.1497, -64.347) (-130.1497, -64.8648) knots 0 0 0 1 1 1
  line L26 (-130.1497, -64.8648) -> (-130.1497, -65.8098)
  line L27 (-130.1497, -65.8098) -> (-131.0551, -65.8098)
  line L28 (-131.0551, -65.8098) -> (-131.0551, -63.6312)
  line L29 (-131.0551, -63.6312) -> (-130.1497, -63.6312)
  line L30 (-130.1497, -63.6312) -> (-130.1497, -64.0132)
  line L31 (-130.1497, -64.0132) -> (-130.1413, -64.0132)
  spline S28 degree 2 poles (-130.1413, -64.0132) (-130.0592, -63.8066) (-129.7508, -63.5916) (-129.5471, -63.5916) knots 0 0 0 1 2 2 2
  spline S29 degree 2 poles (-129.5471, -63.5916) (-129.4735, -63.5916) (-129.417, -63.6171) knots 0 0 0 1 1 1
  line L32 (-129.417, -63.6171) -> (-129.417, -64.4064)
  line L33 (-127.7024, -65.8098) -> (-127.7024, -65.5551)
  line L34 (-127.7024, -65.5551) -> (-127.7109, -65.5551)
  spline S30 degree 2 poles (-127.7109, -65.5551) (-127.8184, -65.6994) (-128.1692, -65.8635) (-128.339, -65.8635) knots 0 0 0 1 2 2 2
  spline S31 degree 2 poles (-128.339, -65.8635) (-128.6163, -65.8635) (-129.0435, -65.5891) (-129.2529, -65.094) (-129.2529, -64.7601) knots 0 0 0 1 2 3 3 3
  spline S32 degree 2 poles (-129.2529, -64.7601) (-129.2529, -64.4121) (-129.001, -63.8745) (-128.5455, -63.5775) (-128.2626, -63.5775) knots 0 0 0 1 2 3 3 3
  spline S33 degree 2 poles (-128.2626, -63.5775) (-128.1296, -63.5775) (-127.9033, -63.6538) (-127.7335, -63.784) (-127.7109, -63.8491) knots 0 0 0 1 2 3 3 3
  line L35 (-127.7109, -63.8491) -> (-127.7024, -63.8491)
  line L36 (-127.7024, -63.8491) -> (-127.7024, -62.5844)
  line L37 (-127.7024, -62.5844) -> (-126.797, -62.5844)
  line L38 (-126.797, -62.5844) -> (-126.797, -65.8098)
  line L39 (-126.797, -65.8098) -> (-127.7024, -65.8098)
  spline S34 degree 2 poles (-127.6826, -64.6554) (-127.6826, -64.4602) (-127.8552, -64.2423) (-128.0023, -64.2423) knots 0 0 0 1 2 2 2
  spline S35 degree 2 poles (-128.0023, -64.2423) (-128.1494, -64.2423) (-128.3333, -64.5111) (-128.3333, -64.7375) knots 0 0 0 1 2 2 2
  spline S36 degree 2 poles (-128.3333, -64.7375) (-128.3333, -65.1987) (-128.0136, -65.1987) knots 0 0 0 1 1 1
  spline S37 degree 2 poles (-128.0136, -65.1987) (-127.8637, -65.1987) (-127.6826, -64.9497) (-127.6826, -64.712) knots 0 0 0 1 2 2 2
  line L40 (-127.6826, -64.712) -> (-127.6826, -64.6554)
  line L41 (-123.0651, -65.8154) -> (-123.2434, -65.6061)
  spline S38 degree 2 poles (-123.2434, -65.6061) (-123.3849, -65.7164) (-123.8998, -65.8635) (-124.1346, -65.8635) knots 0 0 0 1 2 2 2
  spline S39 degree 2 poles (-124.1346, -65.8635) (-124.6552, -65.8635) (-125.2352, -65.4109) (-125.2352, -65.0034) knots 0 0 0 1 2 2 2
  spline S40 degree 2 poles (-125.2352, -65.0034) (-125.2352, -64.7629) (-124.8872, -64.3244) (-124.5279, -64.1461) knots 0 0 0 1 2 2 2
  spline S41 degree 2 poles (-124.5279, -64.1461) (-124.8335, -63.8095) (-124.8335, -63.4756) knots 0 0 0 1 1 1
  spline S42 degree 2 poles (-124.8335, -63.4756) (-124.8335, -63.1333) (-124.2987, -62.7089) (-123.8715, -62.7089) knots 0 0 0 1 2 2 2
  spline S43 degree 2 poles (-123.8715, -62.7089) (-123.4641, -62.7089) (-122.9689, -63.0908) (-122.9689, -63.4077) knots 0 0 0 1 2 2 2
  spline S44 degree 2 poles (-122.9689, -63.4077) (-122.9689, -63.6595) (-123.2632, -64.0245) (-123.5801, -64.1716) knots 0 0 0 1 2 2 2
  line L42 (-123.5801, -64.1716) -> (-123.1472, -64.6639)
  spline S45 degree 2 poles (-123.1472, -64.6639) (-123.051, -64.4715) (-123.051, -64.1461) knots 0 0 0 1 1 1
  line L43 (-123.051, -64.1461) -> (-122.3578, -64.1461)
  spline S46 degree 2 poles (-122.3578, -64.1461) (-122.3578, -64.4545) (-122.5332, -64.9468) (-122.7285, -65.1506) knots 0 0 0 1 2 2 2
  line L44 (-122.7285, -65.1506) -> (-122.1173, -65.8154)
  line L45 (-122.1173, -65.8154) -> (-123.0651, -65.8154)
  spline S47 degree 2 poles (-124.2082, -64.5168) (-124.2987, -64.5592) (-124.4204, -64.7686) (-124.4204, -64.8987) knots 0 0 0 1 2 2 2
  spline S48 degree 2 poles (-124.4204, -64.8987) (-124.4204, -65.0798) (-124.1799, -65.3005) (-124.0045, -65.3005) knots 0 0 0 1 2 2 2
  spline S49 degree 2 poles (-124.0045, -65.3005) (-123.897, -65.3005) (-123.6933, -65.2298) (-123.6253, -65.1732) knots 0 0 0 1 2 2 2
  line L46 (-123.6253, -65.1732) -> (-124.2082, -64.5168)
  spline S50 degree 2 poles (-123.6678, -63.453) (-123.6678, -63.3624) (-123.8008, -63.2323) (-123.8913, -63.2323) knots 0 0 0 1 2 2 2
  spline S51 degree 2 poles (-123.8913, -63.2323) (-123.9988, -63.2323) (-124.1261, -63.3483) (-124.1261, -63.4501) knots 0 0 0 1 2 2 2
  spline S52 degree 2 poles (-124.1261, -63.4501) (-124.1261, -63.5152) (-124.0469, -63.6538) (-123.9054, -63.8151) knots 0 0 0 1 2 2 2
  spline S53 degree 2 poles (-123.9054, -63.8151) (-123.7725, -63.7331) (-123.6678, -63.5633) (-123.6678, -63.453) knots 0 0 0 1 2 2 2
  spline S54 degree 2 poles (-118.3657, -65.7277) (-118.7448, -65.8635) (-119.2399, -65.8635) knots 0 0 0 1 1 1
  spline S55 degree 2 poles (-119.2399, -65.8635) (-119.7266, -65.8635) (-120.4311, -65.4901) (-120.8045, -64.8054) (-120.8045, -64.3555) knots 0 0 0 1 2 3 3 3
  spline S56 degree 2 poles (-120.8045, -64.3555) (-120.8045, -63.8717) (-120.3886, -63.1191) (-119.6275, -62.7089) (-119.1324, -62.7089) knots 0 0 0 1 2 3 3 3
  spline S57 degree 2 poles (-119.1324, -62.7089) (-118.7363, -62.7089) (-118.3657, -62.8051) knots 0 0 0 1 1 1
  line L47 (-118.3657, -62.8051) -> (-118.3657, -63.6538)
  spline S58 degree 2 poles (-118.3657, -63.6538) (-118.493, -63.5775) (-118.8466, -63.4926) (-119.0249, -63.4926) knots 0 0 0 1 2 2 2
  spline S59 degree 2 poles (-119.0249, -63.4926) (-119.4012, -63.4926) (-119.8312, -63.9226) (-119.8312, -64.2904) knots 0 0 0 1 2 2 2
  spline S60 degree 2 poles (-119.8312, -64.2904) (-119.8312, -64.6554) (-119.4012, -65.0798) (-119.039, -65.0798) knots 0 0 0 1 2 2 2
  spline S61 degree 2 poles (-119.039, -65.0798) (-118.7052, -65.0798) (-118.3657, -64.9072) knots 0 0 0 1 1 1
  line L48 (-118.3657, -64.9072) -> (-118.3657, -65.7277)
  line L49 (-116.7643, -65.8098) -> (-116.7643, -65.4788)
  line L50 (-116.7643, -65.4788) -> (-116.7727, -65.4788)
  spline S62 degree 2 poles (-116.7727, -65.4788) (-116.9906, -65.8635) (-117.4376, -65.8635) knots 0 0 0 1 1 1
  spline S63 degree 2 poles (-117.4376, -65.8635) (-117.746, -65.8635) (-118.094, -65.4986) (-118.094, -65.1902) knots 0 0 0 1 2 2 2
  spline S64 degree 2 poles (-118.094, -65.1902) (-118.094, -64.5479) (-117.3047, -64.4461) knots 0 0 0 1 1 1
  line L51 (-117.3047, -64.4461) -> (-116.7643, -64.3753)
  spline S65 degree 2 poles (-116.7643, -64.3753) (-116.7643, -64.2678) (-116.9567, -64.132) (-117.1179, -64.132) knots 0 0 0 1 2 2 2
  spline S66 degree 2 poles (-117.1179, -64.132) (-117.4829, -64.132) (-117.8903, -64.3414) knots 0 0 0 1 1 1
  line L52 (-117.8903, -64.3414) -> (-117.8903, -63.7529)
  spline S67 degree 2 poles (-117.8903, -63.7529) (-117.7149, -63.6765) (-117.1802, -63.5775) (-116.9906, -63.5775) knots 0 0 0 1 2 2 2
  spline S68 degree 2 poles (-116.9906, -63.5775) (-116.4361, -63.5775) (-115.9353, -64.0528) (-115.9353, -64.6073) knots 0 0 0 1 2 2 2
  line L53 (-115.9353, -64.6073) -> (-115.9353, -65.8098)
  line L54 (-115.9353, -65.8098) -> (-116.7643, -65.8098)
  spline S69 degree 2 poles (-117.3018, -65.0685) (-117.3018, -65.1562) (-117.1887, -65.2722) (-117.084, -65.2722) knots 0 0 0 1 2 2 2
  spline S70 degree 2 poles (-117.084, -65.2722) (-116.9425, -65.2722) (-116.7643, -65.06) (-116.7643, -64.8931) knots 0 0 0 1 2 2 2
  line L55 (-116.7643, -64.8931) -> (-116.7643, -64.811)
  line L56 (-116.7643, -64.811) -> (-117.0727, -64.8535)
  spline S71 degree 2 poles (-117.0727, -64.8535) (-117.3018, -64.8931) (-117.3018, -65.0685) knots 0 0 0 1 1 1
  spline S72 degree 2 poles (-113.7567, -65.0855) (-113.7567, -65.4561) (-114.3226, -65.8635) (-114.8262, -65.8635) knots 0 0 0 1 2 2 2
  spline S73 degree 2 poles (-114.8262, -65.8635) (-114.9733, -65.8635) (-115.4062, -65.8041) (-115.542, -65.7617) knots 0 0 0 1 2 2 2
  line L57 (-115.542, -65.7617) -> (-115.542, -65.1251)
  spline S74 degree 2 poles (-115.542, -65.1251) (-115.1402, -65.3033) (-114.8686, -65.3033) knots 0 0 0 1 1 1
  spline S75 degree 2 poles (-114.8686, -65.3033) (-114.6027, -65.3033) (-114.6027, -65.1647) knots 0 0 0 1 1 1
  spline S76 degree 2 poles (-114.6027, -65.1647) (-114.6027, -65.1081) (-114.7272, -65.0317) (-114.9875, -64.9468) knots 0 0 0 1 2 2 2
  spline S77 degree 2 poles (-114.9875, -64.9468) (-115.2789, -64.8535) (-115.542, -64.5507) (-115.542, -64.3102) knots 0 0 0 1 2 2 2
  spline S78 degree 2 poles (-115.542, -64.3102) (-115.542, -63.9707) (-115.0016, -63.5775) (-114.515, -63.5775) knots 0 0 0 1 2 2 2
  spline S79 degree 2 poles (-114.515, -63.5775) (-114.2292, -63.5775) (-113.9095, -63.6595) knots 0 0 0 1 1 1
  line L58 (-113.9095, -63.6595) -> (-113.9095, -64.2706)
  spline S80 degree 2 poles (-113.9095, -64.2706) (-114.0453, -64.2141) (-114.365, -64.1377) (-114.4725, -64.1377) knots 0 0 0 1 2 2 2
  spline S81 degree 2 poles (-114.4725, -64.1377) (-114.5631, -64.1377) (-114.6706, -64.1971) (-114.6706, -64.2508) knots 0 0 0 1 2 2 2
  spline S82 degree 2 poles (-114.6706, -64.2508) (-114.6706, -64.3131) (-114.5546, -64.3895) (-114.382, -64.4432) knots 0 0 0 1 2 2 2
  spline S83 degree 2 poles (-114.382, -64.4432) (-114.0481, -64.5394) (-113.7567, -64.845) (-113.7567, -65.0855) knots 0 0 0 1 2 2 2
  spline S84 degree 2 poles (-112.642, -64.978) (-112.6193, -65.1194) (-112.342, -65.2779) (-112.1157, -65.2779) knots 0 0 0 1 2 2 2
  spline S85 degree 2 poles (-112.1157, -65.2779) (-111.7988, -65.2779) (-111.5159, -65.1562) knots 0 0 0 1 1 1
  line L59 (-111.5159, -65.1562) -> (-111.5159, -65.7306)
  spline S86 degree 2 poles (-111.5159, -65.7306) (-111.8441, -65.8635) (-112.3166, -65.8635) knots 0 0 0 1 1 1
  spline S87 degree 2 poles (-112.3166, -65.8635) (-112.8853, -65.8635) (-113.519, -65.2807) (-113.519, -64.7686) knots 0 0 0 1 2 2 2
  spline S88 degree 2 poles (-113.519, -64.7686) (-113.519, -64.4178) (-113.2418, -63.883) (-112.6957, -63.5775) (-112.3647, -63.5775) knots 0 0 0 1 2 3 3 3
  spline S89 degree 2 poles (-112.3647, -63.5775) (-112.028, -63.5775) (-111.547, -63.8406) (-111.298, -64.3187) (-111.298, -64.6384) knots 0 0 0 1 2 3 3 3
  line L60 (-111.298, -64.6384) -> (-111.298, -64.978)
  line L61 (-111.298, -64.978) -> (-112.642, -64.978)
  spline S90 degree 2 poles (-112.0987, -64.5026) (-112.0987, -64.1263) (-112.3675, -64.1263) knots 0 0 0 1 1 1
  spline S91 degree 2 poles (-112.3675, -64.1263) (-112.4807, -64.1263) (-112.6335, -64.3329) (-112.6476, -64.5026) knots 0 0 0 1 2 2 2
  line L62 (-112.6476, -64.5026) -> (-112.0987, -64.5026)
  spline S92 degree 2 poles (-106.8136, -64.2452) (-106.8136, -64.7092) (-107.204, -65.4222) (-107.9255, -65.8098) (-108.398, -65.8098) knots 0 0 0 1 2 3 3 3
  line L63 (-108.398, -65.8098) -> (-109.691, -65.8098)
  line L64 (-109.691, -65.8098) -> (-109.691, -62.7598)
  line L65 (-109.691, -62.7598) -> (-108.4263, -62.7598)
  spline S93 degree 2 poles (-108.4263, -62.7598) (-106.8136, -62.7598) (-106.8136, -64.2452) knots 0 0 0 1 1 1
  spline S94 degree 2 poles (-107.7897, -64.2537) (-107.7897, -64.033) (-107.9708, -63.6737) (-108.3074, -63.4784) (-108.5338, -63.4784) knots 0 0 0 1 2 3 3 3
  line L66 (-108.5338, -63.4784) -> (-108.7715, -63.4784)
  line L67 (-108.7715, -63.4784) -> (-108.7715, -65.0911)
  line L68 (-108.7715, -65.0911) -> (-108.514, -65.0911)
  spline S95 degree 2 poles (-108.514, -65.0911) (-108.183, -65.0911) (-107.7897, -64.6384) (-107.7897, -64.2537) knots 0 0 0 1 2 2 2
  spline S96 degree 2 poles (-105.6847, -64.978) (-105.662, -65.1194) (-105.3848, -65.2779) (-105.1584, -65.2779) knots 0 0 0 1 2 2 2
  spline S97 degree 2 poles (-105.1584, -65.2779) (-104.8415, -65.2779) (-104.5586, -65.1562) knots 0 0 0 1 1 1
  line L69 (-104.5586, -65.1562) -> (-104.5586, -65.7306)
  spline S98 degree 2 poles (-104.5586, -65.7306) (-104.8868, -65.8635) (-105.3593, -65.8635) knots 0 0 0 1 1 1
  spline S99 degree 2 poles (-105.3593, -65.8635) (-105.928, -65.8635) (-106.5618, -65.2807) (-106.5618, -64.7686) knots 0 0 0 1 2 2 2
  spline S100 degree 2 poles (-106.5618, -64.7686) (-106.5618, -64.4178) (-106.2845, -63.883) (-105.7384, -63.5775) (-105.4074, -63.5775) knots 0 0 0 1 2 3 3 3
  spline S101 degree 2 poles (-105.4074, -63.5775) (-105.0707, -63.5775) (-104.5897, -63.8406) (-104.3407, -64.3187) (-104.3407, -64.6384) knots 0 0 0 1 2 3 3 3
  line L70 (-104.3407, -64.6384) -> (-104.3407, -64.978)
  line L71 (-104.3407, -64.978) -> (-105.6847, -64.978)
  spline S102 degree 2 poles (-105.1414, -64.5026) (-105.1414, -64.1263) (-105.4102, -64.1263) knots 0 0 0 1 1 1
  spline S103 degree 2 poles (-105.4102, -64.1263) (-105.5234, -64.1263) (-105.6762, -64.3329) (-105.6903, -64.5026) knots 0 0 0 1 2 2 2
  line L72 (-105.6903, -64.5026) -> (-105.1414, -64.5026)
  line L73 (-102.4423, -65.8098) -> (-103.5174, -65.8098)
  line L74 (-103.5174, -65.8098) -> (-104.2445, -63.6312)
  line L75 (-104.2445, -63.6312) -> (-103.2996, -63.6312)
  line L76 (-103.2996, -63.6312) -> (-103.0336, -64.8195)
  spline S104 degree 2 poles (-103.0336, -64.8195) (-102.9714, -65.1081) (-102.9629, -65.2524) knots 0 0 0 1 1 1
  line L77 (-102.9629, -65.2524) -> (-102.9516, -65.2524)
  spline S105 degree 2 poles (-102.9516, -65.2524) (-102.9459, -65.21) (-102.9317, -65.1194) (-102.6234, -63.6312) knots 0 0 0 1 2 2 2
  line L78 (-102.6234, -63.6312) -> (-101.684, -63.6312)
  line L79 (-101.684, -63.6312) -> (-102.4423, -65.8098)
  spline S106 degree 2 poles (-100.6853, -64.978) (-100.6626, -65.1194) (-100.3854, -65.2779) (-100.159, -65.2779) knots 0 0 0 1 2 2 2
  spline S107 degree 2 poles (-100.159, -65.2779) (-99.8421, -65.2779) (-99.5592, -65.1562) knots 0 0 0 1 1 1
  line L80 (-99.5592, -65.1562) -> (-99.5592, -65.7306)
  spline S108 degree 2 poles (-99.5592, -65.7306) (-99.8874, -65.8635) (-100.3599, -65.8635) knots 0 0 0 1 1 1
  spline S109 degree 2 poles (-100.3599, -65.8635) (-100.9286, -65.8635) (-101.5624, -65.2807) (-101.5624, -64.7686) knots 0 0 0 1 2 2 2
  spline S110 degree 2 poles (-101.5624, -64.7686) (-101.5624, -64.4178) (-101.2851, -63.883) (-100.739, -63.5775) (-100.408, -63.5775) knots 0 0 0 1 2 3 3 3
  spline S111 degree 2 poles (-100.408, -63.5775) (-100.0713, -63.5775) (-99.5903, -63.8406) (-99.3413, -64.3187) (-99.3413, -64.6384) knots 0 0 0 1 2 3 3 3
  line L81 (-99.3413, -64.6384) -> (-99.3413, -64.978)
  line L82 (-99.3413, -64.978) -> (-100.6853, -64.978)
  spline S112 degree 2 poles (-100.142, -64.5026) (-100.142, -64.1263) (-100.4108, -64.1263) knots 0 0 0 1 1 1
  spline S113 degree 2 poles (-100.4108, -64.1263) (-100.524, -64.1263) (-100.6768, -64.3329) (-100.6909, -64.5026) knots 0 0 0 1 2 2 2
  line L83 (-100.6909, -64.5026) -> (-100.142, -64.5026)
  line L84 (-99.0273, -65.8098) -> (-99.0273, -62.5844)
  line L85 (-99.0273, -62.5844) -> (-98.1219, -62.5844)
  line L86 (-98.1219, -62.5844) -> (-98.1219, -65.8098)
  line L87 (-98.1219, -65.8098) -> (-99.0273, -65.8098)
  spline S114 degree 2 poles (-95.2643, -64.6809) (-95.2643, -65.2326) (-95.9292, -65.8635) (-96.5262, -65.8635) knots 0 0 0 1 2 2 2
  spline S115 degree 2 poles (-96.5262, -65.8635) (-97.1203, -65.8635) (-97.7824, -65.2496) (-97.7824, -64.7064) knots 0 0 0 1 2 2 2
  spline S116 degree 2 poles (-97.7824, -64.7064) (-97.7824, -64.3612) (-97.4712, -63.8491) (-96.8968, -63.5775) (-96.5234, -63.5775) knots 0 0 0 1 2 3 3 3
  spline S117 degree 2 poles (-96.5234, -63.5775) (-96.1357, -63.5775) (-95.567, -63.8632) (-95.2643, -64.3697) (-95.2643, -64.6809) knots 0 0 0 1 2 3 3 3
  spline S118 degree 2 poles (-96.1838, -64.6865) (-96.1838, -64.2423) (-96.5234, -64.2423) knots 0 0 0 1 1 1
  spline S119 degree 2 poles (-96.5234, -64.2423) (-96.8629, -64.2423) (-96.8629, -64.7064) knots 0 0 0 1 1 1
  spline S120 degree 2 poles (-96.8629, -64.7064) (-96.8629, -65.1987) (-96.5177, -65.1987) knots 0 0 0 1 1 1
  spline S121 degree 2 poles (-96.5177, -65.1987) (-96.1838, -65.1987) (-96.1838, -64.6865) knots 0 0 0 1 1 1
  spline S122 degree 2 poles (-92.4689, -64.6554) (-92.4689, -65.0119) (-92.7123, -65.5608) (-93.1536, -65.8635) (-93.4309, -65.8635) knots 0 0 0 1 2 3 3 3
  spline S123 degree 2 poles (-93.4309, -65.8635) (-93.8129, -65.8635) (-94.0109, -65.5834) knots 0 0 0 1 1 1
  line L88 (-94.0109, -65.5834) -> (-94.0194, -65.5834)
  line L89 (-94.0194, -65.5834) -> (-94.0194, -66.8114)
  line L90 (-94.0194, -66.8114) -> (-94.9248, -66.8114)
  line L91 (-94.9248, -66.8114) -> (-94.9248, -63.6312)
  line L92 (-94.9248, -63.6312) -> (-94.0194, -63.6312)
  line L93 (-94.0194, -63.6312) -> (-94.0194, -63.9283)
  line L94 (-94.0194, -63.9283) -> (-94.0109, -63.9283)
  spline S124 degree 2 poles (-94.0109, -63.9283) (-93.9034, -63.7642) (-93.5582, -63.5775) (-93.3375, -63.5775) knots 0 0 0 1 2 2 2
  spline S125 degree 2 poles (-93.3375, -63.5775) (-92.9188, -63.5775) (-92.4689, -64.1405) (-92.4689, -64.6554) knots 0 0 0 1 2 2 2
  spline S126 degree 2 poles (-93.3885, -64.6809) (-93.3885, -64.4772) (-93.5469, -64.2423) (-93.7138, -64.2423) knots 0 0 0 1 2 2 2
  spline S127 degree 2 poles (-93.7138, -64.2423) (-93.8581, -64.2423) (-94.0364, -64.4885) (-94.0364, -64.7035) knots 0 0 0 1 2 2 2
  line L95 (-94.0364, -64.7035) -> (-94.0364, -64.746)
  spline S128 degree 2 poles (-94.0364, -64.746) (-94.0364, -64.9525) (-93.8836, -65.1987) (-93.7308, -65.1987) knots 0 0 0 1 2 2 2
  spline S129 degree 2 poles (-93.7308, -65.1987) (-93.5667, -65.1987) (-93.3885, -64.9299) (-93.3885, -64.6809) knots 0 0 0 1 2 2 2
  spline S130 degree 2 poles (-91.3457, -64.978) (-91.3231, -65.1194) (-91.0458, -65.2779) (-90.8195, -65.2779) knots 0 0 0 1 2 2 2
  spline S131 degree 2 poles (-90.8195, -65.2779) (-90.5026, -65.2779) (-90.2196, -65.1562) knots 0 0 0 1 1 1
  line L96 (-90.2196, -65.1562) -> (-90.2196, -65.7306)
  spline S132 degree 2 poles (-90.2196, -65.7306) (-90.5478, -65.8635) (-91.0203, -65.8635) knots 0 0 0 1 1 1
  spline S133 degree 2 poles (-91.0203, -65.8635) (-91.589, -65.8635) (-92.2228, -65.2807) (-92.2228, -64.7686) knots 0 0 0 1 2 2 2
  spline S134 degree 2 poles (-92.2228, -64.7686) (-92.2228, -64.4178) (-91.9455, -63.883) (-91.3995, -63.5775) (-91.0684, -63.5775) knots 0 0 0 1 2 3 3 3
  spline S135 degree 2 poles (-91.0684, -63.5775) (-90.7317, -63.5775) (-90.2508, -63.8406) (-90.0018, -64.3187) (-90.0018, -64.6384) knots 0 0 0 1 2 3 3 3
  line L97 (-90.0018, -64.6384) -> (-90.0018, -64.978)
  line L98 (-90.0018, -64.978) -> (-91.3457, -64.978)
  spline S136 degree 2 poles (-90.8025, -64.5026) (-90.8025, -64.1263) (-91.0713, -64.1263) knots 0 0 0 1 1 1
  spline S137 degree 2 poles (-91.0713, -64.1263) (-91.1844, -64.1263) (-91.3372, -64.3329) (-91.3514, -64.5026) knots 0 0 0 1 2 2 2
  line L99 (-91.3514, -64.5026) -> (-90.8025, -64.5026)
  line L100 (-88.2335, -65.8098) -> (-88.2335, -65.5551)
  line L101 (-88.2335, -65.5551) -> (-88.242, -65.5551)
  spline S138 degree 2 poles (-88.242, -65.5551) (-88.3495, -65.6994) (-88.7003, -65.8635) (-88.8701, -65.8635) knots 0 0 0 1 2 2 2
  spline S139 degree 2 poles (-88.8701, -65.8635) (-89.1473, -65.8635) (-89.5746, -65.5891) (-89.7839, -65.094) (-89.7839, -64.7601) knots 0 0 0 1 2 3 3 3
  spline S140 degree 2 poles (-89.7839, -64.7601) (-89.7839, -64.4121) (-89.5321, -63.8745) (-89.0766, -63.5775) (-88.7937, -63.5775) knots 0 0 0 1 2 3 3 3
  spline S141 degree 2 poles (-88.7937, -63.5775) (-88.6607, -63.5775) (-88.4343, -63.6538) (-88.2646, -63.784) (-88.242, -63.8491) knots 0 0 0 1 2 3 3 3
  line L102 (-88.242, -63.8491) -> (-88.2335, -63.8491)
  line L103 (-88.2335, -63.8491) -> (-88.2335, -62.5844)
  line L104 (-88.2335, -62.5844) -> (-87.3281, -62.5844)
  line L105 (-87.3281, -62.5844) -> (-87.3281, -65.8098)
  line L106 (-87.3281, -65.8098) -> (-88.2335, -65.8098)
  spline S142 degree 2 poles (-88.2137, -64.6554) (-88.2137, -64.4602) (-88.3862, -64.2423) (-88.5334, -64.2423) knots 0 0 0 1 2 2 2
  spline S143 degree 2 poles (-88.5334, -64.2423) (-88.6805, -64.2423) (-88.8644, -64.5111) (-88.8644, -64.7375) knots 0 0 0 1 2 2 2
  spline S144 degree 2 poles (-88.8644, -64.7375) (-88.8644, -65.1987) (-88.5447, -65.1987) knots 0 0 0 1 1 1
  spline S145 degree 2 poles (-88.5447, -65.1987) (-88.3947, -65.1987) (-88.2137, -64.9497) (-88.2137, -64.712) knots 0 0 0 1 2 2 2
  line L107 (-88.2137, -64.712) -> (-88.2137, -64.6554)
  spline S146 degree 2 poles (-83.2227, -64.6554) (-83.2227, -65.0119) (-83.4576, -65.5636) (-83.8933, -65.8635) (-84.1677, -65.8635) knots 0 0 0 1 2 3 3 3
  spline S147 degree 2 poles (-84.1677, -65.8635) (-84.3771, -65.8635) (-84.677, -65.7079) (-84.7647, -65.5834) knots 0 0 0 1 2 2 2
  line L108 (-84.7647, -65.5834) -> (-84.7732, -65.5834)
  line L109 (-84.7732, -65.5834) -> (-84.7732, -65.8098)
  line L110 (-84.7732, -65.8098) -> (-85.6786, -65.8098)
  line L111 (-85.6786, -65.8098) -> (-85.6786, -62.5844)
  line L112 (-85.6786, -62.5844) -> (-84.7732, -62.5844)
  line L113 (-84.7732, -62.5844) -> (-84.7732, -63.9255)
  line L114 (-84.7732, -63.9255) -> (-84.7647, -63.9255)
  spline S148 degree 2 poles (-84.7647, -63.9255) (-84.6572, -63.7642) (-84.2951, -63.5775) (-84.0744, -63.5775) knots 0 0 0 1 2 2 2